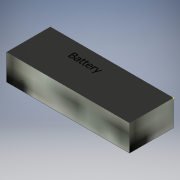
# Autodesk Inventor part: battery
Saved by Autodesk Inventor 2019.4 (Build 234330000, 330)
## iProperties
Created: 2019-06-13
Part Number: battery
Material: Generic
Document SubType Name: Modeling
Designer: abdel
Density: 1 g/cm^3
Appearance: Formwork Holes
Author: abdel
Autodesk Inventor part; units mm, degrees
ref_plane "YZ Plane" through (0, 0, 0) normal (1, 0, 0) x (0, 1, 0)
ref_plane "XZ Plane" through (0, 0, 0) normal (0, 1, 0) x (-1, 0, 0)
ref_plane "XY Plane" through (0, 0, 0) normal (0, 0, 1) x (1, 0, 0)
sketch "Sketch1" plane through (0, 0, 0) normal (0, 1, 0) x (-1, 0, 0)
  line L0 (0, 0) -> (107.95, 0)
  line L1 (107.95, 0) -> (107.95, 38.354)
  line L2 (107.95, 38.354) -> (0, 38.354)
  line L3 (0, 38.354) -> (0, 0)
  dimension "d0" = 107.95
  dimension "d1" = 38.354
  constraints: 8 end point, 2 parallel, 1 horizontal, 1 perpendicular
  measures "d0" distance of L2.end L1.end
  measures "d1" distance of L0.end L1.end
extrude "Extrusion1" add sketch "Sketch1" along normal blind 22.86
sketch "Sketch3" plane through (0, 22.86, 0) normal (0, 1, 0) x (1, 0, 0)
  line L0 (-78.5378, -8.7892) -> (-35.1236, -8.7892) construction
  line L1 (-35.1236, -8.7892) -> (-35.1236, -23.5444) construction
  line L2 (-35.1236, -23.5444) -> (-78.5378, -23.5444) construction
  line L3 (-78.5378, -23.5444) -> (-78.5378, -8.7892) construction
  point P0 (0, 0)
  constraints: 2 other
body "Solid1"
